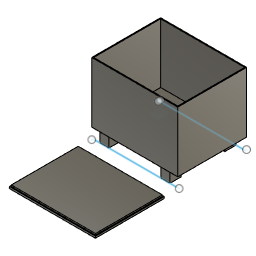
FIRE AND KRISHKA (Autodesk Fusion 360 design; units mm, degrees)
Autodesk Fusion 360 part; units mm, degrees
note: some values were not read from the file. Set by a fixed rule: which face or edge a step refers to.
sketch "Sketch1" plane through (0, 0, 0) normal (0, 0, 1) x (1, 0, 0)
  line L0 (-150, 50) -> (40, 50)
  line L1 (40, 50) -> (40, -102)
  line L2 (40, -102) -> (-150, -102)
  line L3 (-150, -102) -> (-150, 50)
  dimension "d1" = 190
  dimension "d2" = 152
  constraint horizontal L0
  constraint vertical L1
  constraint horizontal L2
  constraint vertical L3
  measures "d1" distance of L0.start L0.end
  measures "d2" distance of L0.start L2.end
extrude "Extrude1" add sketch "Sketch1" along normal blind 3.5 makes body 1
extrude "Extrude2" add 1 faces at (-86.6667, -0.6667, 3.5) along direction (0, 0, 1) blind 130 on bodies 1 bodies 1
shell "Shell1" thickness 2 removed faces 1 at (-86.6667, -0.6667, 133.5) on bodies 1
move_body "Move1" bodies 1 to x (1, 0, 0) y (0, 1, 0) z (0, 0, 1) at (0, 0, 30)
sketch "Sketch2" plane through (0, 0, 30) normal (0, 0, -1) x (1, 0, 0)
  line L0 (40, 102) -> (-150, 102)
  line L1 (-150, 102) -> (-150, -50)
  line L2 (-150, -50) -> (40, -50)
  line L3 (40, -50) -> (40, 102)
  line L4 (-150, 102) -> (-150, 87)
  line L5 (-150, 87) -> (40, 87)
  line L6 (-150, -50) -> (-150, -35)
  line L7 (-150, -35) -> (40, -35)
  line L8 (-135.1928, -35) -> (-115.1928, -35)
  line L9 (-115.1928, -35) -> (-115.1928, -10)
  line L10 (-115.1928, -10) -> (-135.1928, -10)
  line L11 (-135.1928, -10) -> (-135.1928, -35)
  line L12 (-150, -10) -> (40, -10)
  line L13 (-135.1928, -10) -> (-135.1928, 87)
  line L14 (-115.1928, -10) -> (-115.1928, 87)
  line L15 (-135.1928, 87) -> (-115.1928, 87)
  line L16 (-115.1928, 87) -> (-115.1928, 62)
  line L17 (-115.1928, 62) -> (-135.1928, 62)
  line L18 (-135.1928, 62) -> (-135.1928, 87)
  line L19 (-115.1928, 62) -> (40, 62)
  line L20 (-135.1928, 62) -> (-150, 62)
  line L21 (-0.3554, 87) -> (19.6446, 87)
  line L22 (19.6446, 87) -> (19.6446, 62)
  line L23 (19.6446, 62) -> (-0.3554, 62)
  line L24 (-0.3554, 62) -> (-0.3554, 87)
  line L25 (-0.3554, 62) -> (-0.3554, -35)
  line L26 (19.6446, 62) -> (19.6446, -35)
  dimension "d8" = 15
  dimension "d9" = 15
  dimension "d10" = 20
  dimension "d11" = 25
  dimension "d12" = 25
  dimension "d13" = 20
  dimension "d14" = 25
  constraint coincident L0.end L1.start
  constraint coincident L1 L4.end
  constraint coincident L3 L5.end
  constraint perpendicular L3 L5
  constraint coincident L1.end L2.start
  constraint perpendicular L5 L6
  constraint perpendicular L6 L7
  constraint horizontal L8
  constraint vertical L9
  constraint horizontal L10
  constraint vertical L11
  constraint coincident L7 L8.start
  constraint coincident L1 L12.start
  constraint perpendicular L9 L12
  constraint coincident L5 L13.end
  constraint perpendicular L5 L13
  constraint coincident L5 L14.end
  constraint perpendicular L5 L14
  constraint horizontal L15
  constraint vertical L16
  constraint horizontal L17
  constraint vertical L18
  constraint coincident L3 L19.end
  constraint perpendicular L3 L19
  constraint coincident L1 L20.end
  constraint perpendicular L1 L20
  constraint horizontal L21
  constraint vertical L22
  constraint horizontal L23
  constraint vertical L24
  constraint coincident L5 L21.start
  constraint coincident L7 L25.end
  constraint perpendicular L7 L25
  constraint perpendicular L12 L26
  measures "d8" distance of L0.end L4.end
  measures "d9" distance of L1.end L6.end
  measures "d10" distance of L8.start L8.end
  measures "d11" distance of L8.start L10.end
  measures "d12" distance of L13.end L17.end
  measures "d13" distance of L21.start L21.end
  measures "d14" distance of L21.start L23.end
extrude "Extrude3" add sketch "Sketch2" along normal blind 20 contours L5 L19 L21 L22 L23 L24 | L5 L13 L14 L15 L16 L17 L18 | L7 L12 L25 L26 | L7 L8 L9 L10 L11 L12 bodies 1
extrude "Extrude4" add 4 faces at (6.3112, 18.3333, 10) (6.3112, -78.6667, 10) (-128.5261, 18.3333, 10) (-128.5261, -78.6667, 10) along direction (0, 0, -1) blind 4 on bodies 1 bodies 1
sketch "Sketch3" plane through (0, 0, 6) normal (0, 0, -1) x (1, 0, 0)
  line L0 (-135.1928, -10) -> (-135.1928, -35)
  line L1 (-135.1928, -35) -> (-115.1928, -35)
  line L2 (-115.1928, -35) -> (-115.1928, -10)
  line L3 (-115.1928, -10) -> (-135.1928, -10)
  line L4 (-150, -50) -> (-150, -45)
  line L5 (-150, 102) -> (-150, 99)
  line L6 (-150, 99) -> (40, 99)
  line L7 (40, -50) -> (40, -47)
  line L8 (40, -47) -> (-150, -47)
  dimension "d19" = 3
  constraint vertical L4
  constraint vertical L5
  constraint perpendicular L5 L6
  constraint vertical L7
  constraint coincident L4 L8.end
  constraint perpendicular L4 L8
  measures "d19" distance of L7.start L7.end
move_face "MoveFace1" by (0, -12, 0) 10 faces at (-0.3554, -70.3333, 22) (6.3112, -87, 14) (6.3112, -78.6667, 6) (6.3112, -62, 14) (19.6446, -78.6667, 22) (-115.1928, -70.3333, 22) (-128.5261, -87, 14) (-128.5261, -78.6667, 6) (-121.8594, -62, 14) (-135.1928, -70.3333, 22) on bodies 1
move_face "MoveFace2" by (0, 12, 0) 5 faces at (-115.1928, 26.6667, 14) (-128.5261, 35, 14) (-121.8594, 26.6667, 6) (-135.1928, 18.3333, 14) (-121.8594, 10, 14) on bodies 1
move_face "MoveFace3" by (0, 12, 0) 5 faces at (6.3112, 18.3333, 6) (19.6446, 18.3333, 14) (6.3112, 35, 14) (6.3112, 10, 14) (-0.3554, 18.3333, 14) on bodies 1
sketch "Sketch4" plane through (0, 0, 0) normal (0, 0, 1) x (1, 0, 0)
  line L0 (-150, 100) -> (40, 100)
  line L1 (40, 100) -> (40, 252)
  line L2 (40, 252) -> (-150, 252)
  line L3 (-150, 252) -> (-150, 100)
  dimension "d20" = 190
  dimension "d21" = 152
  constraint horizontal L0
  constraint vertical L1
  constraint horizontal L2
  constraint vertical L3
  measures "d20" distance of L0.start L0.end
  measures "d21" distance of L0.start L2.end
extrude "Extrude5" add sketch "Sketch4" along normal blind 4 separate body makes body 2
shell "Shell2" thickness 2 removed faces 1 at (-86.6667, 150.6667, 4) on bodies 2
extrude "Extrude6" add 1 faces at (-86, 200.6667, 2) along direction (0, 0, 1) blind 5 on bodies 2 bodies 2
move_body "Move2" bodies 2 to x (1, 0, 0) y (0, -1, 0) z (0, 0, -1) at (0, 150, 167.5)
move_body "Move3" bodies 2 to x (1, 0, 0) y (0, -1, 0) z (0, 0, -1) at (0, -394, 321)
move_body "Move4" bodies 2 to x (1, 0, 0) y (0, 1, 0) z (0, 0, 1) at (0, 0, -150)
move_body "Move5" bodies 2 to x (1, 0, 0) y (0, 1, 0) z (0, 0, 1) at (0, 160, 0)
